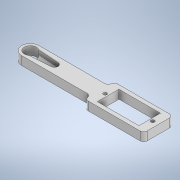
# Autodesk Inventor part: link2
Saved by Autodesk Inventor 2020.2 (Build 242310000, 310)
## iProperties
Created: 2026-05-18
Part Number: link2
Material: Generic
Document SubType Name: Modeling
Designer: explorer
Density: 1 g/cm^3
Appearance: Default
Author: explorer
Autodesk Inventor part; units mm, degrees
ref_plane "YZ Plane" through (0, 0, 0) normal (1, 0, 0) x (0, 1, 0)
ref_plane "XZ Plane" through (0, 0, 0) normal (0, 1, 0) x (-1, 0, 0)
ref_plane "XY Plane" through (0, 0, 0) normal (0, 0, 1) x (1, 0, 0)
sketch "Sketch1" plane through (0, 0, 0) normal (0, 1, 0) x (-1, 0, 0)
  circle A0 centre (0, 0) radius 3.5
  line L0 (0, -5) -> (-40, -5)
  line L1 (-40, -5) -> (-40, 5) construction
  line L2 (-40, 5) -> (0, 5)
  line L3 (0, 5) -> (0, -5) construction
  line L4 (-74, -8.5) -> (-40, -8.5)
  line L5 (-40, -8.5) -> (-40, 8.5)
  line L6 (-40, 8.5) -> (-74, 8.5)
  line L7 (-74, 8.5) -> (-74, -8.5)
  line L8 (20.8, 0) -> (-89.8, 0) projected
  line L9 (0, -11.9) -> (0, 11.9) projected
  arc A1 (0, -5) -> (0, 5) centre (0, 0) ccw
  line L10 (0, 0) -> (0, -5) construction
  line L11 (0, 0) -> (5, 0) construction
  line L12 (0, 0) -> (0, 5) construction
  line L13 (-57, -8.5) -> (-57, 8.5) construction
  line L14 (-45, -6.25) -> (-69, -6.25)
  line L15 (-69, -6.25) -> (-69, 6.25)
  line L16 (-69, 6.25) -> (-45, 6.25)
  line L17 (-45, 6.25) -> (-45, -6.25)
  line L18 (-45, -6.25) -> (-69, 6.25) construction
  line L19 (-69, -6.25) -> (-45, 6.25) construction
  line L20 (-43.25, 0) -> (-70.75, 0) construction
  circle A2 centre (-43.25, 0) radius 1
  circle A3 centre (-70.75, 0) radius 1
  point P0 (-40, 0)
  point P1 (-57, 0)
  point P2 (-57, 0)
  dimension "d0" = 7
  dimension "d2" = 5
  dimension "d3" = 90
  dimension "d4" = 180
  dimension "d5" = 24
  dimension "d6" = 12.5
  dimension "d7" = 17
  dimension "d8" = 34
  dimension "d9" = 2
  dimension "d10" = 27.5
  dimension "d11" = 40
  constraints: 38 end point, 10 midpoint, 5 horizontal, 5 parallel, 4 centre point, 4 coincident, 4 perpendicular, 2 point on circle, 1 equal radius, 1 tangent, 1 vertical
  measures "d0" diameter of A0
  measures "d2" radius of A1
  measures "d3" angle of L10 L11
  measures "d4" angle of L10 L12
  measures "d5" distance of L14.start L14.end
  measures "d6" distance of L14.end L15.end
  measures "d7" distance of L6.end L4.start
  measures "d8" distance of L4.start L4.end
  measures "d9" diameter of A2
  measures "d10" distance of L20.start L20.end
  measures "d11" distance of L1.end L2.end
extrude "Extrusion1" add sketch "Sketch1" along normal blind 5 contours L8 A1 L9 A0 | A0 L9 A1 L8 | A0 L8 L5 L2 L9 | L9 L0 L5 L8 A0 | L8 A2 L17 L16 L15 A3 L7 L6 L5 | L5 L4 L7 L8 A3 L15 L14 L17 A2
sketch "Sketch2" plane through (0, 5, 0) normal (0, 1, 0) x (1, 0, 0)
  circle A0 centre (0, 0) radius 3
  arc A1 (14, -2) -> (14, 2) centre (14, 0) ccw
  line L0 (14, 0) -> (14, 2) construction
  line L1 (14, 0) -> (16, 0) construction
  line L2 (14, 0) -> (14, -2) construction
  line L3 (0, 11.9) -> (0, -11.9) projected
  line L4 (-20.8, 0) -> (89.8, 0) projected
  line L5 (14, 2) -> (0, 3)
  line L6 (14, -2) -> (0, -3)
  dimension "d14" = 6
  dimension "d16" = 90
  dimension "d17" = 180
  dimension "d18" = 14
  dimension "d22" = 2
  constraints: 10 end point, 4 point on circle, 2 centre point, 2 point on line, 1 coincident, 1 horizontal, 1 perpendicular
  measures "d14" diameter of A0
  measures "d16" angle of L1 L0
  measures "d17" angle of L0 L2
  measures "d18" distance of L0.start point (0, 0)
  measures "d22" radius of A1
extrude "Extrusion2" cut sketch "Sketch2" against normal blind 2.5 contours L4 L3 L5 A0 | L4 A1 L6 A0 | A0 L6 L3 L4 | A0 L5 A1 L4 | L4 A0 L3 | L3 A0 L4
fillet "Fillet1" radius 2 6 edges at (40, 2.5, 8.5) (74, 2.5, 8.5) (74, 2.5, -8.5) (40, 2.5, -8.5) (40, 2.5, -5) (40, 2.5, 5)
body "Solid1"
